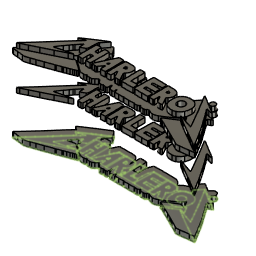
2024_08_12_ZChareloiZlogo v1 (Autodesk Fusion 360 design; units mm, degrees)
Autodesk Fusion 360 part; units mm, degrees
(part 1 of 2)
sketch "Sketch1" plane through (0, 0, 0) normal (0, 0, 1) x (1, 0, 0)
  spline S0 degree 3 poles (34.2287, -11.4604) (33.2659, -10.9653) (32.9545, -10.8069) (32.8689, -10.7687) knots 0 0 0 0 1 1 1 1
  spline S1 degree 3 poles (32.8689, -10.7687) (32.8171, -10.7456) (32.6519, -10.664) (32.5016, -10.5874) knots 0 0 0 0 1 1 1 1
  spline S2 degree 3 poles (32.5016, -10.5874) (32.3514, -10.5107) (32.1873, -10.4304) (32.1371, -10.4088) knots 0 0 0 0 1 1 1 1
  spline S3 degree 3 poles (32.1371, -10.4088) (32.0868, -10.3872) (32.0198, -10.3529) (31.9881, -10.3326) knots 0 0 0 0 1 1 1 1
  spline S4 degree 3 poles (31.9881, -10.3326) (31.9565, -10.3122) (31.5679, -10.1202) (31.1247, -9.9059) knots 0 0 0 0 1 1 1 1
  spline S5 degree 3 poles (31.1247, -9.9059) (30.6815, -9.6916) (30.0228, -9.3715) (29.6609, -9.1945) knots 0 0 0 0 1 1 1 1
  spline S6 degree 3 poles (29.6609, -9.1945) (29.299, -9.0175) (28.994, -8.8728) (28.9831, -8.8728) knots 0 0 0 0 1 1 1 1
  spline S7 degree 3 poles (28.9831, -8.8728) (28.9723, -8.8728) (28.8366, -8.8147) (28.6817, -8.7436) knots 0 0 0 0 1 1 1 1
  spline S8 degree 3 poles (28.6817, -8.7436) (28.5268, -8.6726) (28.3699, -8.6041) (28.3329, -8.5913) knots 0 0 0 0 1 1 1 1
  spline S9 degree 3 poles (28.3329, -8.5913) (28.2382, -8.5587) (28.2493, -8.5074) (28.3713, -8.4142) knots 0 0 0 0 1 1 1 1
  spline S10 degree 3 poles (28.3713, -8.4142) (28.7717, -8.1083) (29.1464, -7.8462) (29.2443, -7.8036) knots 0 0 0 0 1 1 1 1
  spline S11 degree 3 poles (29.2443, -7.8036) (29.3077, -7.776) (29.5063, -7.6576) (29.6857, -7.5404) knots 0 0 0 0 1 1 1 1
  spline S12 degree 3 poles (29.6857, -7.5404) (30.3119, -7.1315) (30.5806, -6.9612) (30.7122, -6.8901) knots 0 0 0 0 1 1 1 1
  spline S13 degree 3 poles (30.7122, -6.8901) (30.7856, -6.8504) (30.855, -6.8632) (31.1727, -6.9746) knots 0 0 0 0 1 1 1 1
  spline S14 degree 3 poles (31.1727, -6.9746) (31.3785, -7.0468) (31.577, -7.1062) (31.614, -7.1067) knots 0 0 0 0 1 1 1 1
  spline S15 degree 3 poles (31.614, -7.1067) (31.7223, -7.108) (31.693, -6.9915) (31.5177, -6.7238) knots 0 0 0 0 1 1 1 1
  spline S16 degree 3 poles (31.5177, -6.7238) (31.4278, -6.5866) (31.2599, -6.3145) (31.1446, -6.119) knots 0 0 0 0 1 1 1 1
  spline S17 degree 3 poles (31.1446, -6.119) (31.0292, -5.9236) (30.9176, -5.7695) (30.8965, -5.7765) knots 0 0 0 0 1 1 1 1
  spline S18 degree 3 poles (30.8965, -5.7765) (30.8753, -5.7836) (30.8081, -5.8744) (30.7471, -5.9783) knots 0 0 0 0 1 1 1 1
  spline S19 degree 3 poles (30.7471, -5.9783) (30.686, -6.0823) (30.566, -6.251) (30.4804, -6.3532) knots 0 0 0 0 1 1 1 1
  spline S20 degree 3 poles (30.4804, -6.3532) (30.1869, -6.7039) (28.4024, -7.9742) (27.6683, -8.355) knots 0 0 0 0 1 1 1 1
  spline S21 degree 3 poles (27.6683, -8.355) (27.2137, -8.5908) (26.9737, -8.6559) (26.6379, -8.6343) knots 0 0 0 0 1 1 1 1
  spline S22 degree 3 poles (26.6379, -8.6343) (26.373, -8.6173) (26.3099, -8.5967) (25.826, -8.3687) knots 0 0 0 0 1 1 1 1
  spline S23 degree 3 poles (25.826, -8.3687) (25.6977, -8.3082) (25.5801, -8.2588) (25.5646, -8.2588) knots 0 0 0 0 1 1 1 1
  spline S24 degree 3 poles (25.5646, -8.2588) (25.5492, -8.2588) (25.4442, -8.3462) (25.3312, -8.453) knots 0 0 0 0 1 1 1 1
  line L0 (25.3312, -8.453) -> (25.1258, -8.6472)
  line L1 (25.1258, -8.6472) -> (24.7867, -8.666)
  spline S25 degree 3 poles (24.7867, -8.666) (24.3803, -8.6884) (24.21, -8.6625) (24.1804, -8.574) knots 0 0 0 0 1 1 1 1
  spline S26 degree 3 poles (24.1804, -8.574) (24.1683, -8.5378) (24.1253, -8.4652) (24.0848, -8.4126) knots 0 0 0 0 1 1 1 1
  line L2 (24.0848, -8.4126) -> (24.0111, -8.317)
  line L3 (24.0111, -8.317) -> (23.8839, -8.462)
  spline S27 degree 3 poles (23.8839, -8.462) (23.7755, -8.5856) (23.7229, -8.6123) (23.5265, -8.6437) knots 0 0 0 0 1 1 1 1
  spline S28 degree 3 poles (23.5265, -8.6437) (23.294, -8.6807) (23.0629, -8.6612) (23.0258, -8.6013) knots 0 0 0 0 1 1 1 1
  spline S29 degree 3 poles (23.0258, -8.6013) (23.0148, -8.5833) (22.962, -8.5853) (22.9087, -8.6056) knots 0 0 0 0 1 1 1 1
  spline S30 degree 3 poles (22.9087, -8.6056) (22.8553, -8.6259) (22.3561, -8.6425) (21.7993, -8.6425) knots 0 0 0 0 1 1 1 1
  spline S31 degree 3 poles (21.7993, -8.6425) (20.8149, -8.6425) (20.7855, -8.6403) (20.7307, -8.562) knots 0 0 0 0 1 1 1 1
  line L4 (20.7307, -8.562) -> (20.6743, -8.4815)
  line L5 (20.6743, -8.4815) -> (20.6308, -8.5627)
  spline S32 degree 3 poles (20.6308, -8.5627) (20.5883, -8.6422) (20.5689, -8.6437) (19.7377, -8.6336) knots 0 0 0 0 1 1 1 1
  line L6 (19.7377, -8.6336) -> (18.8881, -8.6233)
  line L7 (18.8881, -8.6233) -> (18.8352, -8.4314)
  spline S33 degree 3 poles (18.8352, -8.4314) (18.8061, -8.3259) (18.761, -8.163) (18.735, -8.0695) knots 0 0 0 0 1 1 1 1
  spline S34 degree 3 poles (18.735, -8.0695) (18.6734, -7.8483) (18.5859, -7.8096) (18.6128, -8.0154) knots 0 0 0 0 1 1 1 1
  spline S35 degree 3 poles (18.6128, -8.0154) (18.6234, -8.0965) (18.6497, -8.2232) (18.6713, -8.2969) knots 0 0 0 0 1 1 1 1
  spline S36 degree 3 poles (18.6713, -8.2969) (18.7617, -8.6061) (18.7643, -8.6041) (18.2697, -8.6041) knots 0 0 0 0 1 1 1 1
  line L8 (18.2697, -8.6041) -> (17.829, -8.6041)
  line L9 (17.829, -8.6041) -> (17.709, -8.3666)
  spline S37 degree 3 poles (17.709, -8.3666) (17.6431, -8.2359) (17.5649, -8.0503) (17.5353, -7.9541) knots 0 0 0 0 1 1 1 1
  spline S38 degree 3 poles (17.5353, -7.9541) (17.477, -7.7645) (17.3826, -7.6168) (17.3442, -7.6551) knots 0 0 0 0 1 1 1 1
  spline S39 degree 3 poles (17.3442, -7.6551) (17.331, -7.6683) (17.323, -7.8771) (17.3264, -8.1191) knots 0 0 0 0 1 1 1 1
  spline S40 degree 3 poles (17.3264, -8.1191) (17.3306, -8.4295) (17.3187, -8.5676) (17.2856, -8.588) knots 0 0 0 0 1 1 1 1
  spline S41 degree 3 poles (17.2856, -8.588) (17.2599, -8.6039) (17.112, -8.6169) (16.9569, -8.6169) knots 0 0 0 0 1 1 1 1
  spline S42 degree 3 poles (16.9569, -8.6169) (16.7034, -8.6169) (16.6641, -8.6066) (16.5676, -8.5141) knots 0 0 0 0 1 1 1 1
  spline S43 degree 3 poles (16.5676, -8.5141) (16.4573, -8.4084) (16.408, -8.4133) (16.408, -8.5297) knots 0 0 0 0 1 1 1 1
  spline S44 degree 3 poles (16.408, -8.5297) (16.408, -8.6205) (16.3315, -8.6425) (16.0166, -8.6425) knots 0 0 0 0 1 1 1 1
  spline S45 degree 3 poles (16.0166, -8.6425) (15.7138, -8.6425) (15.736, -8.6581) (15.2636, -8.1114) knots 0 0 0 0 1 1 1 1
  spline S46 degree 3 poles (15.2636, -8.1114) (15.0539, -7.8685) (14.96, -7.8276) (14.8681, -7.9387) knots 0 0 0 0 1 1 1 1
  spline S47 degree 3 poles (14.8681, -7.9387) (14.8391, -7.9738) (14.6545, -8.1378) (14.4578, -8.3033) knots 0 0 0 0 1 1 1 1
  line L10 (14.4578, -8.3033) -> (14.1003, -8.6041)
  line L11 (14.1003, -8.6041) -> (13.6629, -8.6041)
  spline S48 degree 3 poles (13.6629, -8.6041) (13.2317, -8.6041) (13.2237, -8.6025) (13.0944, -8.489) knots 0 0 0 0 1 1 1 1
  spline S49 degree 3 poles (13.0944, -8.489) (12.9435, -8.3565) (12.8775, -8.3434) (12.8775, -8.4459) knots 0 0 0 0 1 1 1 1
  spline S50 degree 3 poles (12.8775, -8.4459) (12.8775, -8.559) (12.803, -8.592) (12.4937, -8.6159) knots 0 0 0 0 1 1 1 1
  spline S51 degree 3 poles (12.4937, -8.6159) (11.9706, -8.6564) (11.7736, -8.61) (11.4104, -8.3607) knots 0 0 0 0 1 1 1 1
  spline S52 degree 3 poles (11.4104, -8.3607) (11.2343, -8.2398) (11.0218, -8.0795) (10.9382, -8.0044) knots 0 0 0 0 1 1 1 1
  spline S53 degree 3 poles (10.9382, -8.0044) (10.8545, -7.9293) (10.5388, -7.7024) (10.2366, -7.5001) knots 0 0 0 0 1 1 1 1
  spline S54 degree 3 poles (10.2366, -7.5001) (9.9345, -7.2978) (9.6575, -7.0945) (9.6212, -7.0483) knots 0 0 0 0 1 1 1 1
  spline S55 degree 3 poles (9.6212, -7.0483) (9.5849, -7.0021) (9.5146, -6.9515) (9.4649, -6.9357) knots 0 0 0 0 1 1 1 1
  spline S56 degree 3 poles (9.4649, -6.9357) (9.3766, -6.9077) (9.3751, -6.8994) (9.394, -6.5372) knots 0 0 0 0 1 1 1 1
  spline S57 degree 3 poles (9.394, -6.5372) (9.4046, -6.3338) (9.4065, -6.1483) (9.3981, -6.125) knots 0 0 0 0 1 1 1 1
  spline S58 degree 3 poles (9.3981, -6.125) (9.3872, -6.0949) (9.3405, -6.094) (9.235, -6.1222) knots 0 0 0 0 1 1 1 1
  spline S59 degree 3 poles (9.235, -6.1222) (9.0987, -6.1586) (9.0756, -6.1524) (8.9366, -6.0423) knots 0 0 0 0 1 1 1 1
  spline S60 degree 3 poles (8.9366, -6.0423) (8.8538, -5.9767) (8.7399, -5.9114) (8.6834, -5.8973) knots 0 0 0 0 1 1 1 1
  spline S61 degree 3 poles (8.6834, -5.8973) (8.5649, -5.8675) (8.6112, -5.8208) (8.0013, -6.5854) knots 0 0 0 0 1 1 1 1
  spline S62 degree 3 poles (8.0013, -6.5854) (7.6846, -6.9824) (7.589, -7.1268) (7.6268, -7.1508) knots 0 0 0 0 1 1 1 1
  spline S63 degree 3 poles (7.6268, -7.1508) (7.6948, -7.1939) (7.7066, -7.193) (7.897, -7.1293) knots 0 0 0 0 1 1 1 1
  spline S64 degree 3 poles (7.897, -7.1293) (8.1093, -7.0583) (8.6635, -6.9279) (8.8917, -6.8953) knots 0 0 0 0 1 1 1 1
  spline S65 degree 3 poles (8.8917, -6.8953) (9.1041, -6.8649) (9.136, -6.8797) (9.5965, -7.2218) knots 0 0 0 0 1 1 1 1
  spline S66 degree 3 poles (9.5965, -7.2218) (9.7864, -7.363) (9.9677, -7.4884) (9.9994, -7.5005) knots 0 0 0 0 1 1 1 1
  spline S67 degree 3 poles (9.9994, -7.5005) (10.2234, -7.5864) (11.4017, -8.5219) (11.3505, -8.5731) knots 0 0 0 0 1 1 1 1
  spline S68 degree 3 poles (11.3505, -8.5731) (11.3331, -8.5905) (11.2162, -8.6398) (11.0908, -8.6826) knots 0 0 0 0 1 1 1 1
  spline S69 degree 3 poles (11.0908, -8.6826) (10.9654, -8.7253) (10.8283, -8.7761) (10.7861, -8.7953) knots 0 0 0 0 1 1 1 1
  spline S70 degree 3 poles (10.7861, -8.7953) (10.7439, -8.8145) (10.6143, -8.8673) (10.4983, -8.9125) knots 0 0 0 0 1 1 1 1
  spline S71 degree 3 poles (10.4983, -8.9125) (10.3822, -8.9578) (10.2095, -9.0262) (10.1145, -9.0646) knots 0 0 0 0 1 1 1 1
  spline S72 degree 3 poles (10.1145, -9.0646) (10.0195, -9.103) (9.7864, -9.19) (9.5965, -9.258) knots 0 0 0 0 1 1 1 1
  spline S73 degree 3 poles (9.5965, -9.258) (9.4065, -9.326) (9.1786, -9.4139) (9.0901, -9.4534) knots 0 0 0 0 1 1 1 1
  spline S74 degree 3 poles (9.0901, -9.4534) (9.0015, -9.4928) (8.9152, -9.5252) (8.8982, -9.5253) knots 0 0 0 0 1 1 1 1
  spline S75 degree 3 poles (8.8982, -9.5253) (8.8572, -9.5256) (8.1711, -9.7802) (8.0173, -9.8522) knots 0 0 0 0 1 1 1 1
  spline S76 degree 3 poles (8.0173, -9.8522) (7.9508, -9.8834) (7.8828, -9.9089) (7.8662, -9.9089) knots 0 0 0 0 1 1 1 1
  spline S77 degree 3 poles (7.8662, -9.9089) (7.8385, -9.9089) (6.5138, -10.3823) (6.2003, -10.5043) knots 0 0 0 0 1 1 1 1
  spline S78 degree 3 poles (6.2003, -10.5043) (6.0294, -10.5707) (5.5463, -10.7398) (4.9339, -10.9476) knots 0 0 0 0 1 1 1 1
  spline S79 degree 3 poles (4.9339, -10.9476) (4.6701, -11.0371) (4.2643, -11.1772) (4.0321, -11.2591) knots 0 0 0 0 1 1 1 1
  spline S80 degree 3 poles (4.0321, -11.2591) (3.1935, -11.5545) (3.1144, -11.5705) (2.7274, -11.5234) knots 0 0 0 0 1 1 1 1
  spline S81 degree 3 poles (2.7274, -11.5234) (2.5374, -11.5002) (2.0366, -11.4457) (1.6145, -11.4023) knots 0 0 0 0 1 1 1 1
  spline S82 degree 3 poles (1.6145, -11.4023) (1.1924, -11.3588) (0.7548, -11.3133) (0.6421, -11.3011) knots 0 0 0 0 1 1 1 1
  spline S83 degree 3 poles (0.6421, -11.3011) (0.5186, -11.2877) (0.4291, -11.2576) (0.4166, -11.2251) knots 0 0 0 0 1 1 1 1
  spline S84 degree 3 poles (0.4166, -11.2251) (0.4037, -11.1916) (0.5353, -11.0406) (0.7667, -10.8234) knots 0 0 0 0 1 1 1 1
  spline S85 degree 3 poles (0.7667, -10.8234) (0.9706, -10.6321) (1.3951, -10.1883) (1.7102, -9.8372) knots 0 0 0 0 1 1 1 1
  spline S86 degree 3 poles (1.7102, -9.8372) (2.0252, -9.4862) (2.4434, -9.0256) (2.6395, -8.8136) knots 0 0 0 0 1 1 1 1
  spline S87 degree 3 poles (2.6395, -8.8136) (3.2304, -8.175) (3.6059, -7.7571) (3.8794, -7.4337) knots 0 0 0 0 1 1 1 1
  spline S88 degree 3 poles (3.8794, -7.4337) (4.0222, -7.2649) (4.2535, -6.9972) (4.3933, -6.8389) knots 0 0 0 0 1 1 1 1
  spline S89 degree 3 poles (4.3933, -6.8389) (4.6896, -6.5037) (4.9771, -6.1661) (5.1572, -5.942) knots 0 0 0 0 1 1 1 1
  spline S90 degree 3 poles (5.1572, -5.942) (5.2821, -5.7866) (5.7739, -5.2503) (6.3633, -4.6266) knots 0 0 0 0 1 1 1 1
  spline S91 degree 3 poles (6.3633, -4.6266) (6.5348, -4.4451) (6.6521, -4.2899) (6.6406, -4.2599) knots 0 0 0 0 1 1 1 1
  spline S92 degree 3 poles (6.6406, -4.2599) (6.6296, -4.2312) (6.5131, -4.1496) (6.3817, -4.0785) knots 0 0 0 0 1 1 1 1
  spline S93 degree 3 poles (6.3817, -4.0785) (6.1294, -3.9421) (6.0084, -3.8532) (6.0084, -3.8041) knots 0 0 0 0 1 1 1 1
  spline S94 degree 3 poles (6.0084, -3.8041) (6.0084, -3.7435) (6.5986, -3.3327) (7.9271, -2.4685) knots 0 0 0 0 1 1 1 1
  spline S95 degree 3 poles (7.9271, -2.4685) (8.0432, -2.393) (8.2925, -2.223) (8.4811, -2.0907) knots 0 0 0 0 1 1 1 1
  spline S96 degree 3 poles (8.4811, -2.0907) (8.6697, -1.9584) (8.8384, -1.8502) (8.8561, -1.8502) knots 0 0 0 0 1 1 1 1
  spline S97 degree 3 poles (8.8561, -1.8502) (8.8738, -1.8502) (9.0217, -1.7616) (9.1848, -1.6533) knots 0 0 0 0 1 1 1 1
  spline S98 degree 3 poles (9.1848, -1.6533) (9.5317, -1.423) (9.9097, -1.189) (10.1529, -1.0538) knots 0 0 0 0 1 1 1 1
  spline S99 degree 3 poles (10.1529, -1.0538) (10.2479, -1.0011) (10.3601, -0.9287) (10.4023, -0.8931) knots 0 0 0 0 1 1 1 1
  spline S100 degree 3 poles (10.4023, -0.8931) (10.5375, -0.7788) (10.6853, -0.6989) (10.7614, -0.6989) knots 0 0 0 0 1 1 1 1
  spline S101 degree 3 poles (10.7614, -0.6989) (10.8077, -0.6989) (10.9264, -0.8128) (11.0793, -1.004) knots 0 0 0 0 1 1 1 1
  spline S102 degree 3 poles (11.0793, -1.004) (11.4818, -1.5071) (11.803, -1.956) (11.803, -2.0154) knots 0 0 0 0 1 1 1 1
  spline S103 degree 3 poles (11.803, -2.0154) (11.803, -2.0917) (11.1982, -2.7712) (11.1303, -2.7712) knots 0 0 0 0 1 1 1 1
  spline S104 degree 3 poles (11.1303, -2.7712) (11.1003, -2.7712) (11.0491, -2.823) (11.0163, -2.8863) knots 0 0 0 0 1 1 1 1
  spline S105 degree 3 poles (11.0163, -2.8863) (10.9836, -2.9496) (10.9317, -3.0014) (10.9009, -3.0014) knots 0 0 0 0 1 1 1 1
  spline S106 degree 3 poles (10.9009, -3.0014) (10.8702, -3.0014) (10.8341, -3.0453) (10.8206, -3.0989) knots 0 0 0 0 1 1 1 1
  spline S107 degree 3 poles (10.8206, -3.0989) (10.789, -3.2248) (10.9261, -3.5919) (11.0109, -3.6086) knots 0 0 0 0 1 1 1 1
  spline S108 degree 3 poles (11.0109, -3.6086) (11.0653, -3.6193) (11.0739, -3.5768) (11.0739, -3.2967) knots 0 0 0 0 1 1 1 1
  spline S109 degree 3 poles (11.0739, -3.2967) (11.0739, -3.0836) (11.0903, -2.9591) (11.1218, -2.9336) knots 0 0 0 0 1 1 1 1
  spline S110 degree 3 poles (11.1218, -2.9336) (11.1815, -2.8853) (12.0616, -2.8306) (12.2113, -2.8658) knots 0 0 0 0 1 1 1 1
  spline S111 degree 3 poles (12.2113, -2.8658) (12.319, -2.8912) (12.4289, -3.0221) (13.0736, -3.8933) knots 0 0 0 0 1 1 1 1
  spline S112 degree 3 poles (13.0736, -3.8933) (13.2918, -4.1881) (13.3968, -4.2648) (13.4736, -4.1852) knots 0 0 0 0 1 1 1 1
  spline S113 degree 3 poles (13.4736, -4.1852) (13.501, -4.1567) (13.6225, -3.9176) (13.7436, -3.6538) knots 0 0 0 0 1 1 1 1
  spline S114 degree 3 poles (13.7436, -3.6538) (13.8646, -3.39) (14.0092, -3.105) (14.0648, -3.0206) knots 0 0 0 0 1 1 1 1
  line L12 (14.0648, -3.0206) -> (14.166, -2.8671)
  line L13 (14.166, -2.8671) -> (15.6995, -2.8671)
  spline S115 degree 3 poles (15.6995, -2.8671) (17.2186, -2.8671) (17.2353, -2.868) (17.472, -2.9578) knots 0 0 0 0 1 1 1 1
  spline S116 degree 3 poles (17.472, -2.9578) (17.9033, -3.1215) (18.1384, -3.46) (18.2087, -4.0186) knots 0 0 0 0 1 1 1 1
  spline S117 degree 3 poles (18.2087, -4.0186) (18.304, -4.7762) (18.3209, -4.8888) (18.3426, -4.9104) knots 0 0 0 0 1 1 1 1
  spline S118 degree 3 poles (18.3426, -4.9104) (18.3753, -4.9432) (18.3801, -4.8092) (18.3823, -3.8009) knots 0 0 0 0 1 1 1 1
  spline S119 degree 3 poles (18.3823, -3.8009) (18.3834, -3.3015) (18.3986, -2.8784) (18.4161, -2.8608) knots 0 0 0 0 1 1 1 1
  spline S120 degree 3 poles (18.4161, -2.8608) (18.4692, -2.8075) (19.6276, -2.797) (19.6906, -2.8492) knots 0 0 0 0 1 1 1 1
  spline S121 degree 3 poles (19.6906, -2.8492) (19.7353, -2.8863) (19.745, -3.0972) (19.7452, -4.032) knots 0 0 0 0 1 1 1 1
  spline S122 degree 3 poles (19.7452, -4.032) (19.7453, -4.6577) (19.7566, -5.2938) (19.7703, -5.4457) knots 0 0 0 0 1 1 1 1
  line L14 (19.7703, -5.4457) -> (19.7952, -5.7218)
  line L15 (19.7952, -5.7218) -> (20.0063, -5.7482)
  spline S123 degree 3 poles (20.0063, -5.7482) (20.2149, -5.7742) (20.6975, -5.7472) (20.7375, -5.7072) knots 0 0 0 0 1 1 1 1
  spline S124 degree 3 poles (20.7375, -5.7072) (20.7489, -5.6959) (20.7651, -5.3026) (20.7737, -4.8333) knots 0 0 0 0 1 1 1 1
  spline S125 degree 3 poles (20.7737, -4.8333) (20.7877, -4.0596) (20.7977, -3.9549) (20.8804, -3.7113) knots 0 0 0 0 1 1 1 1
  spline S126 degree 3 poles (20.8804, -3.7113) (21.0886, -3.0982) (21.169, -2.9029) (21.2329, -2.856) knots 0 0 0 0 1 1 1 1
  spline S127 degree 3 poles (21.2329, -2.856) (21.3254, -2.7881) (25.6254, -2.8122) (25.8865, -2.8821) knots 0 0 0 0 1 1 1 1
  spline S128 degree 3 poles (25.8865, -2.8821) (26.3826, -3.0148) (26.8083, -3.3765) (26.8985, -3.7418) knots 0 0 0 0 1 1 1 1
  spline S129 degree 3 poles (26.8985, -3.7418) (26.913, -3.8007) (26.948, -3.8578) (26.9761, -3.8686) knots 0 0 0 0 1 1 1 1
  spline S130 degree 3 poles (26.9761, -3.8686) (27.0057, -3.8799) (27.1716, -3.7446) (27.3683, -3.5486) knots 0 0 0 0 1 1 1 1
  spline S131 degree 3 poles (27.3683, -3.5486) (27.646, -3.2721) (27.77, -3.1799) (28.0355, -3.0523) knots 0 0 0 0 1 1 1 1
  spline S132 degree 3 poles (28.0355, -3.0523) (28.3202, -2.9155) (28.4557, -2.8725) (28.8702, -2.7874) knots 0 0 0 0 1 1 1 1
  spline S133 degree 3 poles (28.8702, -2.7874) (28.9177, -2.7777) (28.9565, -2.7558) (28.9565, -2.7388) knots 0 0 0 0 1 1 1 1
  spline S134 degree 3 poles (28.9565, -2.7388) (28.9565, -2.7218) (28.8615, -2.581) (28.7455, -2.4258) knots 0 0 0 0 1 1 1 1
  spline S135 degree 3 poles (28.7455, -2.4258) (28.6294, -2.2706) (28.5344, -2.1183) (28.5344, -2.0873) knots 0 0 0 0 1 1 1 1
  spline S136 degree 3 poles (28.5344, -2.0873) (28.5344, -2.0562) (28.6078, -1.95) (28.6975, -1.8511) knots 0 0 0 0 1 1 1 1
  spline S137 degree 3 poles (28.6975, -1.8511) (28.7872, -1.7523) (28.921, -1.5895) (28.9949, -1.4894) knots 0 0 0 0 1 1 1 1
  spline S138 degree 3 poles (28.9949, -1.4894) (29.2185, -1.1862) (29.5757, -0.7713) (29.6315, -0.7499) knots 0 0 0 0 1 1 1 1
  spline S139 degree 3 poles (29.6315, -0.7499) (29.6923, -0.7265) (30.0084, -0.8977) (30.6834, -1.3196) knots 0 0 0 0 1 1 1 1
  spline S140 degree 3 poles (30.6834, -1.3196) (30.9472, -1.4845) (31.1912, -1.6196) (31.2256, -1.6197) knots 0 0 0 0 1 1 1 1
  spline S141 degree 3 poles (31.2256, -1.6197) (31.26, -1.6198) (31.3488, -1.5465) (31.4228, -1.4568) knots 0 0 0 0 1 1 1 1
  spline S142 degree 3 poles (31.4228, -1.4568) (31.78, -1.0244) (31.8676, -0.9671) (32.1691, -0.9688) knots 0 0 0 0 1 1 1 1
  spline S143 degree 3 poles (32.1691, -0.9688) (32.5579, -0.9711) (32.8265, -1.237) (32.8305, -1.6236) knots 0 0 0 0 1 1 1 1
  spline S144 degree 3 poles (32.8305, -1.6236) (32.8329, -1.8532) (32.7538, -2.0048) (32.5333, -2.1933) knots 0 0 0 0 1 1 1 1
  spline S145 degree 3 poles (32.5333, -2.1933) (32.3203, -2.3753) (32.2732, -2.3218) (33.0252, -2.752) knots 0 0 0 0 1 1 1 1
  spline S146 degree 3 poles (33.0252, -2.752) (33.7119, -3.1448) (34.0796, -3.3905) (34.0796, -3.4567) knots 0 0 0 0 1 1 1 1
  spline S147 degree 3 poles (34.0796, -3.4567) (34.0796, -3.4855) (33.9469, -3.5804) (33.7848, -3.6677) knots 0 0 0 0 1 1 1 1
  spline S148 degree 3 poles (33.7848, -3.6677) (33.6227, -3.755) (33.443, -3.8616) (33.3857, -3.9045) knots 0 0 0 0 1 1 1 1
  spline S149 degree 3 poles (33.3857, -3.9045) (33.2638, -3.9957) (33.2665, -4.004) (33.5569, -4.4346) knots 0 0 0 0 1 1 1 1
  spline S150 degree 3 poles (33.5569, -4.4346) (33.6544, -4.5792) (33.7514, -4.726) (33.7726, -4.7608) knots 0 0 0 0 1 1 1 1
  spline S151 degree 3 poles (33.7726, -4.7608) (33.7937, -4.7957) (33.8196, -4.8329) (33.8301, -4.8434) knots 0 0 0 0 1 1 1 1
  spline S152 degree 3 poles (33.8301, -4.8434) (33.8407, -4.854) (33.9261, -4.9748) (34.02, -5.112) knots 0 0 0 0 1 1 1 1
  spline S153 degree 3 poles (34.02, -5.112) (34.1138, -5.2492) (34.2008, -5.3701) (34.2132, -5.3807) knots 0 0 0 0 1 1 1 1
  spline S154 degree 3 poles (34.2132, -5.3807) (34.2256, -5.3912) (34.2998, -5.4948) (34.3782, -5.6109) knots 0 0 0 0 1 1 1 1
  spline S155 degree 3 poles (34.3782, -5.6109) (34.5845, -5.9165) (34.7313, -6.123) (35.0193, -6.5127) knots 0 0 0 0 1 1 1 1
  spline S156 degree 3 poles (35.0193, -6.5127) (35.1597, -6.7027) (35.3438, -6.9617) (35.4284, -7.0883) knots 0 0 0 0 1 1 1 1
  spline S157 degree 3 poles (35.4284, -7.0883) (35.513, -7.215) (35.6939, -7.4826) (35.8304, -7.6831) knots 0 0 0 0 1 1 1 1
  spline S158 degree 3 poles (35.8304, -7.6831) (35.9668, -7.8836) (36.1454, -8.1599) (36.2272, -8.2971) knots 0 0 0 0 1 1 1 1
  spline S159 degree 3 poles (36.2272, -8.2971) (36.309, -8.4343) (36.6584, -8.9998) (37.0037, -9.5537) knots 0 0 0 0 1 1 1 1
  spline S160 degree 3 poles (37.0037, -9.5537) (37.349, -10.1076) (37.6422, -10.5911) (37.6554, -10.6282) knots 0 0 0 0 1 1 1 1
  spline S161 degree 3 poles (37.6554, -10.6282) (37.6685, -10.6652) (37.7053, -10.7259) (37.7372, -10.763) knots 0 0 0 0 1 1 1 1
  spline S162 degree 3 poles (37.7372, -10.763) (37.8432, -10.8864) (37.9897, -11.1729) (37.9613, -11.2013) knots 0 0 0 0 1 1 1 1
  spline S163 degree 3 poles (37.9613, -11.2013) (37.9343, -11.2283) (37.5489, -11.2887) (37.0344, -11.3465) knots 0 0 0 0 1 1 1 1
  spline S164 degree 3 poles (37.0344, -11.3465) (36.5443, -11.4016) (36.0491, -11.4656) (35.25, -11.5771) knots 0 0 0 0 1 1 1 1
  spline S165 degree 3 poles (35.25, -11.5771) (34.6469, -11.6612) (34.6113, -11.6572) (34.2287, -11.4604) knots 0 0 0 0 1 1 1 1
  spline S166 degree 3 poles (37.6676, -10.99) (37.6676, -10.9725) (37.6189, -10.8818) (37.5593, -10.7885) knots 0 0 0 0 1 1 1 1
  spline S167 degree 3 poles (37.5593, -10.7885) (37.4998, -10.6952) (37.338, -10.4289) (37.1999, -10.1967) knots 0 0 0 0 1 1 1 1
  spline S168 degree 3 poles (37.1999, -10.1967) (36.8471, -9.6039) (36.3337, -8.7671) (36.2111, -8.5849) knots 0 0 0 0 1 1 1 1
  spline S169 degree 3 poles (36.2111, -8.5849) (36.1543, -8.5005) (36.0474, -8.3365) (35.9736, -8.2204) knots 0 0 0 0 1 1 1 1
  spline S170 degree 3 poles (35.9736, -8.2204) (35.5846, -7.6086) (34.7351, -6.345) (34.4644, -5.9755) knots 0 0 0 0 1 1 1 1
  spline S171 degree 3 poles (34.4644, -5.9755) (34.2943, -5.7433) (34.0621, -5.4152) (33.9483, -5.2463) knots 0 0 0 0 1 1 1 1
  spline S172 degree 3 poles (33.9483, -5.2463) (33.8346, -5.0775) (33.6779, -4.853) (33.6002, -4.7475) knots 0 0 0 0 1 1 1 1
  spline S173 degree 3 poles (33.6002, -4.7475) (33.5225, -4.6419) (33.3258, -4.3743) (33.1631, -4.1527) knots 0 0 0 0 1 1 1 1
  spline S174 degree 3 poles (33.1631, -4.1527) (33.0005, -3.931) (32.7861, -3.647) (32.6868, -3.5215) knots 0 0 0 0 1 1 1 1
  spline S175 degree 3 poles (32.6868, -3.5215) (32.4749, -3.2537) (32.393, -3.1165) (32.4451, -3.1165) knots 0 0 0 0 1 1 1 1
  spline S176 degree 3 poles (32.4451, -3.1165) (32.4656, -3.1165) (32.6863, -3.166) (32.9356, -3.2265) knots 0 0 0 0 1 1 1 1
  spline S177 degree 3 poles (32.9356, -3.2265) (33.469, -3.356) (33.7535, -3.402) (33.7531, -3.3587) knots 0 0 0 0 1 1 1 1
  spline S178 degree 3 poles (33.7531, -3.3587) (33.7528, -3.316) (33.5954, -3.2137) (32.9475, -2.8355) knots 0 0 0 0 1 1 1 1
  spline S179 degree 3 poles (32.9475, -2.8355) (32.3996, -2.5156) (32.1934, -2.3914) (31.6619, -2.0613) knots 0 0 0 0 1 1 1 1
  spline S180 degree 3 poles (31.6619, -2.0613) (30.1943, -1.1497) (29.9305, -0.9947) (29.8772, -1.0124) knots 0 0 0 0 1 1 1 1
  spline S181 degree 3 poles (29.8772, -1.0124) (29.8545, -1.02) (29.9529, -1.2072) (30.0957, -1.4286) knots 0 0 0 0 1 1 1 1
  spline S182 degree 3 poles (30.0957, -1.4286) (30.3967, -1.8952) (30.7393, -2.4548) (31.1877, -3.2125) knots 0 0 0 0 1 1 1 1
  spline S183 degree 3 poles (31.1877, -3.2125) (31.3626, -3.508) (31.5981, -3.8939) (31.7112, -4.0701) knots 0 0 0 0 1 1 1 1
  spline S184 degree 3 poles (31.7112, -4.0701) (31.8242, -4.2462) (31.9272, -4.4189) (31.94, -4.4538) knots 0 0 0 0 1 1 1 1
  spline S185 degree 3 poles (31.94, -4.4538) (31.9528, -4.4887) (32.0066, -4.5863) (32.0595, -4.6707) knots 0 0 0 0 1 1 1 1
  spline S186 degree 3 poles (32.0595, -4.6707) (32.1473, -4.8108) (32.2714, -5.0236) (32.5069, -5.4382) knots 0 0 0 0 1 1 1 1
  spline S187 degree 3 poles (32.5069, -5.4382) (32.5549, -5.5226) (32.7686, -5.8918) (32.9819, -6.2586) knots 0 0 0 0 1 1 1 1
  spline S188 degree 3 poles (32.9819, -6.2586) (33.1951, -6.6253) (33.3696, -6.931) (33.3696, -6.9379) knots 0 0 0 0 1 1 1 1
  spline S189 degree 3 poles (33.3696, -6.9379) (33.3696, -6.9447) (33.4876, -7.1541) (33.6317, -7.4031) knots 0 0 0 0 1 1 1 1
  spline S190 degree 3 poles (33.6317, -7.4031) (33.9063, -7.8774) (33.9609, -7.9905) (33.9153, -7.9896) knots 0 0 0 0 1 1 1 1
  spline S191 degree 3 poles (33.9153, -7.9896) (33.8503, -7.9883) (32.8668, -7.6829) (32.6213, -7.5877) knots 0 0 0 0 1 1 1 1
  spline S192 degree 3 poles (32.6213, -7.5877) (32.3302, -7.4749) (31.0111, -7.0308) (30.9671, -7.0308) knots 0 0 0 0 1 1 1 1
  spline S193 degree 3 poles (30.9671, -7.0308) (30.9522, -7.0308) (30.9714, -7.0653) (31.0096, -7.1075) knots 0 0 0 0 1 1 1 1
  spline S194 degree 3 poles (31.0096, -7.1075) (31.0478, -7.1497) (31.0924, -7.1843) (31.1086, -7.1843) knots 0 0 0 0 1 1 1 1
  spline S195 degree 3 poles (31.1086, -7.1843) (31.1249, -7.1843) (31.2647, -7.2676) (31.4193, -7.3695) knots 0 0 0 0 1 1 1 1
  spline S196 degree 3 poles (31.4193, -7.3695) (31.5739, -7.4714) (31.8267, -7.6312) (31.9813, -7.7245) knots 0 0 0 0 1 1 1 1
  spline S197 degree 3 poles (31.9813, -7.7245) (32.1358, -7.8178) (32.3028, -7.9201) (32.3524, -7.9518) knots 0 0 0 0 1 1 1 1
  spline S198 degree 3 poles (32.3524, -7.9518) (32.6698, -8.1544) (34.5483, -9.2565) (34.5763, -9.2565) knots 0 0 0 0 1 1 1 1
  spline S199 degree 3 poles (34.5763, -9.2565) (34.5865, -9.2565) (34.7639, -9.3545) (34.9704, -9.4743) knots 0 0 0 0 1 1 1 1
  spline S200 degree 3 poles (34.9704, -9.4743) (35.1769, -9.5941) (35.3891, -9.7156) (35.4419, -9.7442) knots 0 0 0 0 1 1 1 1
  spline S201 degree 3 poles (35.4419, -9.7442) (35.4946, -9.7728) (35.7796, -9.9438) (36.075, -10.1241) knots 0 0 0 0 1 1 1 1
  spline S202 degree 3 poles (36.075, -10.1241) (36.3705, -10.3044) (36.7332, -10.5181) (36.8809, -10.5989) knots 0 0 0 0 1 1 1 1
  spline S203 degree 3 poles (36.8809, -10.5989) (37.0287, -10.6797) (37.2521, -10.8079) (37.3775, -10.8838) knots 0 0 0 0 1 1 1 1
  spline S204 degree 3 poles (37.3775, -10.8838) (37.6109, -11.025) (37.6676, -11.0458) (37.6676, -10.99) knots 0 0 0 0 1 1 1 1
  spline S205 degree 3 poles (1.358, -10.735) (1.5835, -10.6195) (2.1306, -10.3494) (2.5739, -10.1348) knots 0 0 0 0 1 1 1 1
  spline S206 degree 3 poles (2.5739, -10.1348) (3.0171, -9.9202) (3.7338, -9.5732) (4.1664, -9.3639) knots 0 0 0 0 1 1 1 1
  spline S207 degree 3 poles (4.1664, -9.3639) (4.5991, -9.1545) (5.4884, -8.7179) (6.1427, -8.3937) knots 0 0 0 0 1 1 1 1
  spline S208 degree 3 poles (6.1427, -8.3937) (6.797, -8.0695) (7.6757, -7.6383) (8.0953, -7.4353) knots 0 0 0 0 1 1 1 1
  spline S209 degree 3 poles (8.0953, -7.4353) (8.5149, -7.2324) (8.8501, -7.0583) (8.8402, -7.0484) knots 0 0 0 0 1 1 1 1
  spline S210 degree 3 poles (8.8402, -7.0484) (8.8169, -7.0251) (7.3943, -7.362) (6.3922, -7.6283) knots 0 0 0 0 1 1 1 1
  spline S211 degree 3 poles (6.3922, -7.6283) (5.5847, -7.8429) (5.4712, -7.8639) (5.4712, -7.7992) knots 0 0 0 0 1 1 1 1
  spline S212 degree 3 poles (5.4712, -7.7992) (5.4712, -7.752) (5.9191, -7.0848) (6.264, -6.6182) knots 0 0 0 0 1 1 1 1
  spline S213 degree 3 poles (6.264, -6.6182) (6.4084, -6.4229) (6.6387, -6.1072) (6.7759, -5.9165) knots 0 0 0 0 1 1 1 1
  spline S214 degree 3 poles (6.7759, -5.9165) (6.9131, -5.7259) (7.0653, -5.5144) (7.1141, -5.4465) knots 0 0 0 0 1 1 1 1
  spline S215 degree 3 poles (7.1141, -5.4465) (7.163, -5.3786) (7.2407, -5.2796) (7.2868, -5.2265) knots 0 0 0 0 1 1 1 1
  spline S216 degree 3 poles (7.2868, -5.2265) (7.5615, -4.9102) (7.7805, -4.6439) (7.9252, -4.4501) knots 0 0 0 0 1 1 1 1
  spline S217 degree 3 poles (7.9252, -4.4501) (8.0158, -4.3287) (8.1051, -4.2294) (8.1236, -4.2294) knots 0 0 0 0 1 1 1 1
  spline S218 degree 3 poles (8.1236, -4.2294) (8.1422, -4.2294) (8.1574, -4.4539) (8.1574, -4.7283) knots 0 0 0 0 1 1 1 1
  spline S219 degree 3 poles (8.1574, -4.7283) (8.1574, -5.1458) (8.1668, -5.2272) (8.2149, -5.2272) knots 0 0 0 0 1 1 1 1
  spline S220 degree 3 poles (8.2149, -5.2272) (8.2703, -5.2272) (8.8216, -4.9338) (9.1188, -4.7462) knots 0 0 0 0 1 1 1 1
  spline S221 degree 3 poles (9.1188, -4.7462) (9.304, -4.6293) (9.3096, -4.5942) (9.3267, -3.4475) knots 0 0 0 0 1 1 1 1
  line L16 (9.3267, -3.4475) -> (9.3402, -2.5371)
  line L17 (9.3402, -2.5371) -> (9.478, -2.3759)
  spline S222 degree 3 poles (9.478, -2.3759) (9.7609, -2.0451) (10.5422, -1.037) (10.5273, -1.0222) knots 0 0 0 0 1 1 1 1
  spline S223 degree 3 poles (10.5273, -1.0222) (10.5071, -1.002) (9.8343, -1.4047) (9.2402, -1.7926) knots 0 0 0 0 1 1 1 1
  spline S224 degree 3 poles (9.2402, -1.7926) (8.9816, -1.9615) (8.5243, -2.2588) (8.2239, -2.4534) knots 0 0 0 0 1 1 1 1
  spline S225 degree 3 poles (8.2239, -2.4534) (7.5856, -2.8668) (6.6151, -3.5363) (6.4497, -3.6771) knots 0 0 0 0 1 1 1 1
  spline S226 degree 3 poles (6.4497, -3.6771) (6.3383, -3.7721) (6.3377, -3.7744) (6.4305, -3.7485) knots 0 0 0 0 1 1 1 1
  spline S227 degree 3 poles (6.4305, -3.7485) (6.4833, -3.7338) (6.7855, -3.6224) (7.1021, -3.5009) knots 0 0 0 0 1 1 1 1
  spline S228 degree 3 poles (7.1021, -3.5009) (7.4187, -3.3795) (7.6833, -3.2944) (7.69, -3.312) knots 0 0 0 0 1 1 1 1
  spline S229 degree 3 poles (7.69, -3.312) (7.7, -3.3379) (7.2467, -3.8925) (7.1597, -3.9608) knots 0 0 0 0 1 1 1 1
  spline S230 degree 3 poles (7.1597, -3.9608) (7.0592, -4.0397) (5.1843, -6.1253) (4.4159, -7.013) knots 0 0 0 0 1 1 1 1
  spline S231 degree 3 poles (4.4159, -7.013) (3.3271, -8.2709) (2.0576, -9.6742) (1.3209, -10.4343) knots 0 0 0 0 1 1 1 1
  spline S232 degree 3 poles (1.3209, -10.4343) (0.953, -10.8139) (0.8517, -10.945) (0.9263, -10.945) knots 0 0 0 0 1 1 1 1
  spline S233 degree 3 poles (0.9263, -10.945) (0.9383, -10.945) (1.1325, -10.8505) (1.358, -10.735) knots 0 0 0 0 1 1 1 1
  spline S234 degree 3 poles (10.5611, -6.8581) (10.5757, -6.7948) (10.5906, -6.4494) (10.5941, -6.0906) knots 0 0 0 0 1 1 1 1
  spline S235 degree 3 poles (10.5941, -6.0906) (10.5977, -5.7318) (10.6034, -5.4159) (10.607, -5.3886) knots 0 0 0 0 1 1 1 1
  spline S236 degree 3 poles (10.607, -5.3886) (10.6117, -5.3518) (10.69, -5.3419) (10.9108, -5.3503) knots 0 0 0 0 1 1 1 1
  line L18 (10.9108, -5.3503) -> (11.2082, -5.3615)
  line L19 (11.2082, -5.3615) -> (11.2103, -6.0522)
  spline S237 degree 3 poles (11.2103, -6.0522) (11.2114, -6.4321) (11.2157, -6.7904) (11.2199, -6.8485) knots 0 0 0 0 1 1 1 1
  line L20 (11.2199, -6.8485) -> (11.2274, -6.954)
  line L21 (11.2274, -6.954) -> (11.6836, -6.954)
  line L22 (11.6836, -6.954) -> (12.1398, -6.954)
  line L23 (12.1398, -6.954) -> (12.1652, -6.0618)
  spline S238 degree 3 poles (12.1652, -6.0618) (12.2026, -4.7472) (12.21, -3.089) (12.1785, -3.0573) knots 0 0 0 0 1 1 1 1
  spline S239 degree 3 poles (12.1785, -3.0573) (12.1367, -3.0152) (11.6405, -2.9883) (11.4455, -3.0175) knots 0 0 0 0 1 1 1 1
  spline S240 degree 3 poles (11.4455, -3.0175) (11.3504, -3.0318) (11.2637, -3.0666) (11.2528, -3.095) knots 0 0 0 0 1 1 1 1
  spline S241 degree 3 poles (11.2528, -3.095) (11.2419, -3.1233) (11.2207, -3.4333) (11.2055, -3.7839) knots 0 0 0 0 1 1 1 1
  line L24 (11.2055, -3.7839) -> (11.178, -4.4213)
  line L25 (11.178, -4.4213) -> (10.8998, -4.4213)
  spline S242 degree 3 poles (10.8998, -4.4213) (10.6798, -4.4213) (10.6167, -4.4084) (10.598, -4.3597) knots 0 0 0 0 1 1 1 1
  spline S243 degree 3 poles (10.598, -4.3597) (10.585, -4.3258) (10.5761, -4.0223) (10.5783, -3.6853) knots 0 0 0 0 1 1 1 1
  spline S244 degree 3 poles (10.5783, -3.6853) (10.5804, -3.3483) (10.5735, -3.0638) (10.5628, -3.0531) knots 0 0 0 0 1 1 1 1
  spline S245 degree 3 poles (10.5628, -3.0531) (10.5202, -3.0106) (9.6195, -3.0211) (9.5757, -3.0647) knots 0 0 0 0 1 1 1 1
  spline S246 degree 3 poles (9.5757, -3.0647) (9.5275, -3.1126) (9.5173, -6.0385) (9.5633, -6.6356) knots 0 0 0 0 1 1 1 1
  line L26 (9.5633, -6.6356) -> (9.5875, -6.9504)
  line L27 (9.5875, -6.9504) -> (9.7839, -6.962)
  spline S247 degree 3 poles (9.7839, -6.962) (9.8919, -6.9685) (10.1049, -6.9736) (10.2574, -6.9735) knots 0 0 0 0 1 1 1 1
  spline S248 degree 3 poles (10.2574, -6.9735) (10.5338, -6.9732) (10.5346, -6.9729) (10.5611, -6.8581) knots 0 0 0 0 1 1 1 1
  spline S249 degree 3 poles (15.2567, -6.9191) (15.2814, -6.9147) (15.2724, -5.1158) (15.2421, -3.9992) knots 0 0 0 0 1 1 1 1
  spline S250 degree 3 poles (15.2421, -3.9992) (15.2292, -3.5243) (15.2186, -3.1055) (15.2185, -3.0686) knots 0 0 0 0 1 1 1 1
  spline S251 degree 3 poles (15.2185, -3.0686) (15.2184, -3.008) (15.1685, -3.0014) (14.7094, -3.0014) knots 0 0 0 0 1 1 1 1
  line L28 (14.7094, -3.0014) -> (14.2004, -3.0014)
  line L29 (14.2004, -3.0014) -> (14.0599, -3.2796)
  spline S252 degree 3 poles (14.0599, -3.2796) (13.8054, -3.7834) (13.425, -4.586) (13.2095, -5.0737) knots 0 0 0 0 1 1 1 1
  spline S253 degree 3 poles (13.2095, -5.0737) (13.0929, -5.3375) (12.8608, -5.8555) (12.6937, -6.2249) knots 0 0 0 0 1 1 1 1
  line L30 (12.6937, -6.2249) -> (12.39, -6.8965)
  line L31 (12.39, -6.8965) -> (12.5282, -6.923)
  spline S254 degree 3 poles (12.5282, -6.923) (12.6042, -6.9376) (12.8305, -6.9501) (13.031, -6.9506) knots 0 0 0 0 1 1 1 1
  line L32 (13.031, -6.9506) -> (13.3956, -6.9517)
  line L33 (13.3956, -6.9517) -> (13.5153, -6.7897)
  spline S255 degree 3 poles (13.5153, -6.7897) (13.5812, -6.7007) (13.7642, -6.451) (13.9219, -6.2349) knots 0 0 0 0 1 1 1 1
  spline S256 degree 3 poles (13.9219, -6.2349) (14.0796, -6.0188) (14.22, -5.8533) (14.2338, -5.8672) knots 0 0 0 0 1 1 1 1
  spline S257 degree 3 poles (14.2338, -5.8672) (14.2477, -5.881) (14.259, -6.1298) (14.259, -6.42) knots 0 0 0 0 1 1 1 1
  spline S258 degree 3 poles (14.259, -6.42) (14.259, -6.7341) (14.2744, -6.9528) (14.297, -6.9604) knots 0 0 0 0 1 1 1 1
  spline S259 degree 3 poles (14.297, -6.9604) (14.3267, -6.9704) (15.1736, -6.934) (15.2567, -6.9191) knots 0 0 0 0 1 1 1 1
  spline S260 degree 3 poles (14.0286, -5.1984) (14.1548, -4.9756) (14.2119, -4.9103) (14.2564, -4.9378) knots 0 0 0 0 1 1 1 1
  spline S261 degree 3 poles (14.2564, -4.9378) (14.3013, -4.9655) (14.3095, -5.1205) (14.2732, -5.2559) knots 0 0 0 0 1 1 1 1
  spline S262 degree 3 poles (14.2732, -5.2559) (14.2541, -5.327) (14.2232, -5.3423) (14.0986, -5.3423) knots 0 0 0 0 1 1 1 1
  line L34 (14.0986, -5.3423) -> (13.9471, -5.3423)
  line L35 (13.9471, -5.3423) -> (14.0286, -5.1984)
  spline S263 degree 3 poles (16.4336, -6.9412) (16.4511, -6.9236) (16.4595, -6.6171) (16.4521, -6.26) knots 0 0 0 0 1 1 1 1
  spline S264 degree 3 poles (16.4521, -6.26) (16.4429, -5.8155) (16.4515, -5.6109) (16.4798, -5.6109) knots 0 0 0 0 1 1 1 1
  spline S265 degree 3 poles (16.4798, -5.6109) (16.5024, -5.6109) (16.6708, -5.911) (16.854, -6.2778) knots 0 0 0 0 1 1 1 1
  line L36 (16.854, -6.2778) -> (17.1871, -6.9447)
  line L37 (17.1871, -6.9447) -> (17.3828, -6.9682)
  spline S266 degree 3 poles (17.3828, -6.9682) (17.4904, -6.9812) (17.7314, -6.9919) (17.9183, -6.9921) knots 0 0 0 0 1 1 1 1
  line L38 (17.9183, -6.9921) -> (18.2583, -6.9924)
  line L39 (18.2583, -6.9924) -> (18.2324, -6.8892)
  spline S267 degree 3 poles (18.2324, -6.8892) (18.2181, -6.8325) (18.1757, -6.7418) (18.1382, -6.6877) knots 0 0 0 0 1 1 1 1
  spline S268 degree 3 poles (18.1382, -6.6877) (18.1006, -6.6337) (17.9215, -6.3028) (17.7401, -5.9524) knots 0 0 0 0 1 1 1 1
  line L40 (17.7401, -5.9524) -> (17.4104, -5.3153)
  line L41 (17.4104, -5.3153) -> (17.5774, -5.1514)
  spline S269 degree 3 poles (17.5774, -5.1514) (18.0043, -4.7324) (18.1751, -3.9554) (17.9411, -3.4966) knots 0 0 0 0 1 1 1 1
  spline S270 degree 3 poles (17.9411, -3.4966) (17.85, -3.3181) (17.5648, -3.0938) (17.3522, -3.0335) knots 0 0 0 0 1 1 1 1
  spline S271 degree 3 poles (17.3522, -3.0335) (17.1877, -2.9868) (15.9321, -2.9781) (15.6726, -3.0217) knots 0 0 0 0 1 1 1 1
  line L42 (15.6726, -3.0217) -> (15.5321, -3.0454)
  line L43 (15.5321, -3.0454) -> (15.5052, -3.4038)
  spline S272 degree 3 poles (15.5052, -3.4038) (15.4607, -3.9975) (15.5035, -6.9168) (15.5572, -6.95) knots 0 0 0 0 1 1 1 1
  spline S273 degree 3 poles (15.5572, -6.95) (15.6198, -6.9887) (16.3938, -6.9809) (16.4336, -6.9412) knots 0 0 0 0 1 1 1 1
  spline S274 degree 3 poles (16.46, -4.3631) (16.4477, -4.3311) (16.4495, -4.2102) (16.464, -4.0945) knots 0 0 0 0 1 1 1 1
  line L44 (16.464, -4.0945) -> (16.4903, -3.884)
  line L45 (16.4903, -3.884) -> (16.6358, -3.884)
  spline S275 degree 3 poles (16.6358, -3.884) (16.9287, -3.884) (17.0912, -4.1602) (16.9069, -4.3445) knots 0 0 0 0 1 1 1 1
  spline S276 degree 3 poles (16.9069, -4.3445) (16.8105, -4.4409) (16.4949, -4.454) (16.46, -4.3631) knots 0 0 0 0 1 1 1 1
  spline S277 degree 3 poles (20.9918, -6.9488) (21.03, -6.9084) (21.035, -5.989) (20.9972, -5.9644) knots 0 0 0 0 1 1 1 1
  spline S278 degree 3 poles (20.9972, -5.9644) (20.9742, -5.9494) (20.6446, -5.9371) (20.2646, -5.9371) knots 0 0 0 0 1 1 1 1
  line L46 (20.2646, -5.9371) -> (19.5739, -5.9371)
  line L47 (19.5739, -5.9371) -> (19.5505, -4.4788)
  spline S279 degree 3 poles (19.5505, -4.4788) (19.5377, -3.6768) (19.5247, -3.0114) (19.5217, -3.0002) knots 0 0 0 0 1 1 1 1
  spline S280 degree 3 poles (19.5217, -3.0002) (19.5135, -2.9692) (19.1105, -2.9619) (18.7912, -2.9868) knots 0 0 0 0 1 1 1 1
  line L48 (18.7912, -2.9868) -> (18.5073, -3.009)
  line L49 (18.5073, -3.009) -> (18.5317, -4.1852)
  spline S281 degree 3 poles (18.5317, -4.1852) (18.5451, -4.8322) (18.5563, -5.7187) (18.5565, -6.1554) knots 0 0 0 0 1 1 1 1
  line L50 (18.5565, -6.1554) -> (18.557, -6.9494)
  line L51 (18.557, -6.9494) -> (18.7009, -6.9623)
  spline S282 degree 3 poles (18.7009, -6.9623) (18.8893, -6.9792) (20.9748, -6.9669) (20.9918, -6.9488) knots 0 0 0 0 1 1 1 1
  spline S283 degree 3 poles (24.0932, -6.5525) (24.1051, -6.3105) (24.1063, -6.0798) (24.0958, -6.0398) knots 0 0 0 0 1 1 1 1
  spline S284 degree 3 poles (24.0958, -6.0398) (24.0717, -5.9476) (23.7678, -5.9179) (22.8473, -5.9179) knots 0 0 0 0 1 1 1 1
  line L52 (22.8473, -5.9179) -> (22.1989, -5.9179)
  line L53 (22.1989, -5.9179) -> (22.2103, -5.6781)
  line L54 (22.2103, -5.6781) -> (22.2218, -5.4382)
  line L55 (22.2218, -5.4382) -> (23.1524, -5.4279)
  line L56 (23.1524, -5.4279) -> (24.0829, -5.4177)
  line L57 (24.0829, -5.4177) -> (24.0829, -4.9195)
  line L58 (24.0829, -4.9195) -> (24.0829, -4.4213)
  line L59 (24.0829, -4.4213) -> (23.167, -4.4213)
  line L60 (23.167, -4.4213) -> (22.251, -4.4213)
  line L61 (22.251, -4.4213) -> (22.2283, -4.2816)
  spline S285 degree 3 poles (22.2283, -4.2816) (22.1837, -4.0063) (22.1733, -4.0094) (23.1489, -4.003) knots 0 0 0 0 1 1 1 1
  spline S286 degree 3 poles (23.1489, -4.003) (23.6285, -3.9998) (24.0303, -3.9878) (24.0418, -3.9763) knots 0 0 0 0 1 1 1 1
  spline S287 degree 3 poles (24.0418, -3.9763) (24.0742, -3.944) (24.0624, -3.0448) (24.0292, -3.0116) knots 0 0 0 0 1 1 1 1
  spline S288 degree 3 poles (24.0292, -3.0116) (24.013, -2.9955) (23.3901, -2.9761) (22.645, -2.9687) knots 0 0 0 0 1 1 1 1
  line L62 (22.645, -2.9687) -> (21.2902, -2.9551)
  line L63 (21.2902, -2.9551) -> (21.2642, -3.621)
  spline S289 degree 3 poles (21.2642, -3.621) (21.2186, -4.79) (21.1836, -6.7006) (21.2056, -6.8197) knots 0 0 0 0 1 1 1 1
  spline S290 degree 3 poles (21.2056, -6.8197) (21.225, -6.9252) (21.2427, -6.9367) (21.4173, -6.9576) knots 0 0 0 0 1 1 1 1
  spline S291 degree 3 poles (21.4173, -6.9576) (21.522, -6.9701) (22.1621, -6.9831) (22.8397, -6.9864) knots 0 0 0 0 1 1 1 1
  line L64 (22.8397, -6.9864) -> (24.0715, -6.9924)
  line L65 (24.0715, -6.9924) -> (24.0932, -6.5525)
  line L66 (25.1254, -6.969) -> (25.296, -6.9456)
  line L67 (25.296, -6.9456) -> (25.2947, -6.7867)
  spline S292 degree 3 poles (25.2947, -6.7867) (25.2939, -6.6993) (25.2974, -6.4126) (25.3021, -6.1495) knots 0 0 0 0 1 1 1 1
  spline S293 degree 3 poles (25.3021, -6.1495) (25.3127, -5.5649) (25.3093, -5.5632) (25.717, -6.3592) knots 0 0 0 0 1 1 1 1
  spline S294 degree 3 poles (25.717, -6.3592) (26.057, -7.0231) (26.0017, -6.9863) (26.6635, -6.9902) knots 0 0 0 0 1 1 1 1
  spline S295 degree 3 poles (26.6635, -6.9902) (26.9795, -6.9921) (27.0377, -6.983) (27.0377, -6.9319) knots 0 0 0 0 1 1 1 1
  spline S296 degree 3 poles (27.0377, -6.9319) (27.0377, -6.8638) (26.656, -6.1328) (26.379, -5.6705) knots 0 0 0 0 1 1 1 1
  line L68 (26.379, -5.6705) -> (26.1962, -5.3655)
  line L69 (26.1962, -5.3655) -> (26.4076, -5.1439)
  spline S297 degree 3 poles (26.4076, -5.1439) (26.7058, -4.8312) (26.7834, -4.6394) (26.785, -4.2102) knots 0 0 0 0 1 1 1 1
  spline S298 degree 3 poles (26.785, -4.2102) (26.7866, -3.7908) (26.7316, -3.6179) (26.5257, -3.3946) knots 0 0 0 0 1 1 1 1
  spline S299 degree 3 poles (26.5257, -3.3946) (26.2068, -3.0486) (25.874, -2.9675) (24.7608, -2.9644) knots 0 0 0 0 1 1 1 1
  line L70 (24.7608, -2.9644) -> (24.2684, -2.963)
  line L71 (24.2684, -2.963) -> (24.2817, -4.9487)
  line L72 (24.2817, -4.9487) -> (24.295, -6.9343)
  line L73 (24.295, -6.9343) -> (24.4096, -6.9588)
  spline S300 degree 3 poles (24.4096, -6.9588) (24.5661, -6.9923) (24.9188, -6.9973) (25.1254, -6.969) knots 0 0 0 0 1 1 1 1
  spline S301 degree 3 poles (25.25, -4.3687) (25.2389, -4.3398) (25.2351, -4.2233) (25.2416, -4.1097) knots 0 0 0 0 1 1 1 1
  spline S302 degree 3 poles (25.2416, -4.1097) (25.252, -3.9262) (25.2634, -3.9018) (25.3436, -3.8905) knots 0 0 0 0 1 1 1 1
  spline S303 degree 3 poles (25.3436, -3.8905) (25.5942, -3.855) (25.7778, -4.0288) (25.6966, -4.2247) knots 0 0 0 0 1 1 1 1
  spline S304 degree 3 poles (25.6966, -4.2247) (25.6266, -4.3937) (25.3, -4.4991) (25.25, -4.3687) knots 0 0 0 0 1 1 1 1
  spline S305 degree 3 poles (29.6794, -6.7628) (30.0731, -6.5576) (30.415, -6.2187) (30.5873, -5.8626) knots 0 0 0 0 1 1 1 1
  spline S306 degree 3 poles (30.5873, -5.8626) (30.7322, -5.5634) (30.8364, -4.9785) (30.8201, -4.5556) knots 0 0 0 0 1 1 1 1
  spline S307 degree 3 poles (30.8201, -4.5556) (30.778, -3.4581) (29.6502, -2.7201) (28.468, -3.0165) knots 0 0 0 0 1 1 1 1
  spline S308 degree 3 poles (28.468, -3.0165) (27.9921, -3.1358) (27.5342, -3.4681) (27.3327, -3.8404) knots 0 0 0 0 1 1 1 1
  spline S309 degree 3 poles (27.3327, -3.8404) (27.1541, -4.1705) (27.0985, -4.4375) (27.1, -4.9585) knots 0 0 0 0 1 1 1 1
  spline S310 degree 3 poles (27.1, -4.9585) (27.1024, -5.7753) (27.2588, -6.2416) (27.6325, -6.546) knots 0 0 0 0 1 1 1 1
  spline S311 degree 3 poles (27.6325, -6.546) (28.0286, -6.8687) (28.382, -6.9654) (29.0463, -6.9327) knots 0 0 0 0 1 1 1 1
  spline S312 degree 3 poles (29.0463, -6.9327) (29.3504, -6.9177) (29.4158, -6.9002) (29.6794, -6.7628) knots 0 0 0 0 1 1 1 1
  spline S313 degree 3 poles (28.5536, -5.5915) (28.2864, -5.4471) (28.1118, -5.152) (28.1125, -4.846) knots 0 0 0 0 1 1 1 1
  spline S314 degree 3 poles (28.1125, -4.846) (28.1135, -4.3169) (28.5919, -3.9698) (29.1184, -4.116) knots 0 0 0 0 1 1 1 1
  spline S315 degree 3 poles (29.1184, -4.116) (29.7051, -4.2789) (29.8331, -5.1103) (29.3328, -5.5081) knots 0 0 0 0 1 1 1 1
  spline S316 degree 3 poles (29.3328, -5.5081) (29.215, -5.6018) (29.147, -5.6236) (28.9299, -5.6373) knots 0 0 0 0 1 1 1 1
  spline S317 degree 3 poles (28.9299, -5.6373) (28.737, -5.6495) (28.6386, -5.6375) (28.5536, -5.5915) knots 0 0 0 0 1 1 1 1
  spline S318 degree 3 poles (18.3989, -6.2153) (18.4026, -5.9404) (18.393, -5.8795) (18.3459, -5.8795) knots 0 0 0 0 1 1 1 1
  spline S319 degree 3 poles (18.3459, -5.8795) (18.3142, -5.8795) (18.2883, -5.895) (18.2883, -5.9138) knots 0 0 0 0 1 1 1 1
  spline S320 degree 3 poles (18.2883, -5.9138) (18.2883, -5.9327) (18.2354, -6.0048) (18.1707, -6.0741) knots 0 0 0 0 1 1 1 1
  spline S321 degree 3 poles (18.1707, -6.0741) (18.0345, -6.2199) (18.0386, -6.2623) (18.2189, -6.5703) knots 0 0 0 0 1 1 1 1
  line L74 (18.2189, -6.5703) -> (18.3426, -6.7813)
  line L75 (18.3426, -6.7813) -> (18.3685, -6.6662)
  spline S322 degree 3 poles (18.3685, -6.6662) (18.3827, -6.6029) (18.3964, -6.4) (18.3989, -6.2153) knots 0 0 0 0 1 1 1 1
  spline S323 degree 3 poles (32.3797, -2.1556) (32.548, -2.1089) (32.6627, -1.9759) (32.7208, -1.7603) knots 0 0 0 0 1 1 1 1
  spline S324 degree 3 poles (32.7208, -1.7603) (32.8403, -1.3164) (32.4457, -0.9772) (31.9835, -1.1265) knots 0 0 0 0 1 1 1 1
  spline S325 degree 3 poles (31.9835, -1.1265) (31.7548, -1.2004) (31.6649, -1.3381) (31.6633, -1.6173) knots 0 0 0 0 1 1 1 1
  spline S326 degree 3 poles (31.6633, -1.6173) (31.6622, -1.8132) (31.6775, -1.8621) (31.7806, -1.9895) knots 0 0 0 0 1 1 1 1
  spline S327 degree 3 poles (31.7806, -1.9895) (31.9395, -2.186) (32.1051, -2.2319) (32.3797, -2.1556) knots 0 0 0 0 1 1 1 1
extrude "Extrude1" add sketch "Sketch1" along normal blind 1 contours S166 S167 S168 S169 S170 S171 S172 S173 S174 S175 S176 S177 S178 S179 S180 S181 S182 S183 S184 S185 S186 S187 S188 S189 S190 S191 S192 S193 S194 S195 S196 S197 S198 S199 S200 S201 S202 S203 S204 | S205 S206 S207 S208 S209 S210 S211 S212 S213 S214 S215 S216 S217 S218 S219 S220 S221 L16 L17 S222 S223 S224 S225 S226 S227 S228 S229 S230 S231 S232 S233 | S234 S235 S236 L18 L19 S237 L20 L21 L22 L23 S238 S239 S240 S241 L24 L25 S242 S243 S244 S245 S246 L26 L27 S247 S248 | S249 S250 S251 L28 L29 S252 S253 L30 L31 S254 L32 L33 S255 S256 S257 S258 S259 | S263 S264 S265 L36 L37 S266 L38 L39 S267 S268 L40 L41 S269 S270 S271 L42 L43 S272 S273 | S277 S278 L46 L47 S279 S280 L48 L49 S281 L50 L51 S282 | S283 S284 L52 L53 L54 L55 L56 L57 L58 L59 L60 L61 S285 S286 S287 S288 L62 L63 S289 S290 S291 L64 L65 | L66 L67 S292 S293 S294 S295 S296 L68 L69 S297 S298 S299 L70 L71 L72 L73 S300 | S305 S306 S307 S308 S309 S310 S311 S312 makes body 1 at (24.6263, -6.0108, 0) makes body 2 at (14.5145, -4.0703, 0) makes body 3 at (11.8406, -4.5135, 0) makes body 4 at (21.5638, -5.293, 0) makes body 5 at (27.4619, -5.1984, 0) makes body 6 at (15.8426, -5.3294, 0) makes body 7 at (4.6845, -8.0587, 0) makes body 8 at (19.7556, -6.6161, 0) makes body 9 at (34.772, -7.3463, 0)
move_body "Move1" bodies 9 8 5 2 1 3 6 4 7 to x (1, 0, 0) y (0, 1, 0) z (0, 0, 1) at (0, 0, 8)
extrude "Extrude2" add sketch "Sketch1" against normal blind 1 separate body contours S0 S1 S2 S3 S4 S5 S6 S7 S8 S9 S10 S11 S12 S13 S14 S15 S16 S17 S18 S19 S20 S21 S22 S23 S24 L0 L1 S25 S26 L2 L3 S27 S28 S29 S30 S31 L4 L5 S32 L6 L7 S33 S34 S35 S36 L8 L9 S37 S38 S39 S40 S41 S42 S43 S44 S45 S46 S47 L10 L11 S48 S49 S50 S51 S52 S53 S54 S55 S56 S57 S58 S59 S60 S61 S62 S63 S64 S65 S66 S67 S68 S69 S70 S71 S72 S73 S74 S75 S76 S77 S78 S79 S80 S81 S82 S83 S84 S85 S86 S87 S88 S89 S90 S91 S92 S93 S94 S95 S96 S97 S98 S99 S100 S101 S102 S103 S104 S105 S106 S107 S108 S109 S110 S111 S112 S113 S114 L12 L13 S115 S116 S117 S118 S119 S120 S121 S122 L14 L15 S123 S124 S125 S126 S127 S128 S129 S130 S131 S132 S133 S134 S135 S136 S137 S138 S139 S140 S141 S142 S143 S144 S145 S146 S147 S148 S149 S150 S151 S152 S153 S154 S155 S156 S157 S158 S159 S160 S161 S162 S163 S164 S165 | S166 S167 S168 S169 S170 S171 S172 S173 S174 S175 S176 S177 S178 S179 S180 S181 S182 S183 S184 S185 S186 S187 S188 S189 S190 S191 S192 S193 S194 S195 S196 S197 S198 S199 S200 S201 S202 S203 S204 | S205 S206 S207 S208 S209 S210 S211 S212 S213 S214 S215 S216 S217 S218 S219 S220 S221 L16 L17 S222 S223 S224 S225 S226 S227 S228 S229 S230 S231 S232 S233 | S234 S235 S236 L18 L19 S237 L20 L21 L22 L23 S238 S239 S240 S241 L24 L25 S242 S243 S244 S245 S246 L26 L27 S247 S248 | S249 S250 S251 L28 L29 S252 S253 L30 L31 S254 L32 L33 S255 S256 S257 S258 S259 | S263 S264 S265 L36 L37 S266 L38 L39 S267 S268 L40 L41 S269 S270 S271 L42 L43 S272 S273 | S277 S278 L46 L47 S279 S280 L48 L49 S281 L50 L51 S282 | S283 S284 L52 L53 L54 L55 L56 L57 L58 L59 L60 L61 S285 S286 S287 S288 L62 L63 S289 S290 S291 L64 L65 | L66 L67 S292 S293 S294 S295 S296 L68 L69 S297 S298 S299 L70 L71 L72 L73 S300 | S305 S306 S307 S308 S309 S310 S311 S312 | S318 S319 S320 S321 L74 L75 S322 | S323 S324 S325 S326 S327 makes body 10
extrude "Extrude3" add sketch "Sketch1" along normal blind 1 contours S166 S167 S168 S169 S170 S171 S172 S173 S174 S175 S176 S177 S178 S179 S180 S181 S182 S183 S184 S185 S186 S187 S188 S189 S190 S191 S192 S193 S194 S195 S196 S197 S198 S199 S200 S201 S202 S203 S204 | S205 S206 S207 S208 S209 S210 S211 S212 S213 S214 S215 S216 S217 S218 S219 S220 S221 L16 L17 S222 S223 S224 S225 S226 S227 S228 S229 S230 S231 S232 S233 | S234 S235 S236 L18 L19 S237 L20 L21 L22 L23 S238 S239 S240 S241 L24 L25 S242 S243 S244 S245 S246 L26 L27 S247 S248 | S249 S250 S251 L28 L29 S252 S253 L30 L31 S254 L32 L33 S255 S256 S257 S258 S259 | S263 S264 S265 L36 L37 S266 L38 L39 S267 S268 L40 L41 S269 S270 S271 L42 L43 S272 S273 | S277 S278 L46 L47 S279 S280 L48 L49 S281 L50 L51 S282 | S283 S284 L52 L53 L54 L55 L56 L57 L58 L59 L60 L61 S285 S286 S287 S288 L62 L63 S289 S290 S291 L64 L65 | L66 L67 S292 S293 S294 S295 S296 L68 L69 S297 S298 S299 L70 L71 L72 L73 S300 | S305 S306 S307 S308 S309 S310 S311 S312 | S323 S324 S325 S326 S327 bodies 10